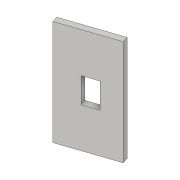
# Autodesk Inventor part: Lidar Sensor Case Piece 4
Saved by Autodesk Inventor 2018.3 (Build 223284000, 284)
## iProperties
Created: 2019-02-26
Part Number: Lidar Sensor Case Piece 4
Material: Generic
Document SubType Name: Modeling
Designer: aye06091
Mass: 4.13207 g
Surface Area: 33.6312 cm^2
Volume: 4.13207 cm^3
Density: 1 g/cm^3
Appearance: Default
Author: aye06091
Autodesk Inventor part; units mm, degrees
ref_plane "YZ Plane" through (0, 0, 0) normal (1, 0, 0) x (0, 1, 0)
ref_plane "XZ Plane" through (0, 0, 0) normal (0, 1, 0) x (-1, 0, 0)
ref_plane "XY Plane" through (0, 0, 0) normal (0, 0, 1) x (1, 0, 0)
sketch "Sketch1" plane through (0, 0, 0) normal (0, 1, 0) x (-1, 0, 0)
  line L0 (1.0684, 9.7831) -> (-25.4217, 0.8993)
  line L1 (-26.3747, 3.741) -> (0.1154, 12.6248)
  line L2 (1.0684, 9.7831) -> (0.1154, 12.6248)
  line L3 (-25.4217, 0.8993) -> (-26.3747, 3.741)
  point P0 (0, 0)
  point P1 (-9.2456, 5.0352)
  dimension "d0" = 27.94
  dimension "d5" = 2.9972
  constraints: 8 end point
  measures "d0" distance of L0.start L0.end
  measures "d5" distance between parallel lines of L1 L0
extrude "Extrusion1" add sketch "Sketch1" along normal blind 52.8066
sketch "Sketch2" plane through (-1.0684, 0, 9.7831) normal (-0.318, 0, -0.9481) x (-0.9481, 0, 0.318)
  line L0 (0, 0) -> (-27.94, 0) projected
  line L1 (-27.94, 52.8066) -> (0, 52.8066) projected
  line L2 (-18.7775, 20.0533) -> (-11.1575, 20.0533)
  line L3 (-11.1575, 20.0533) -> (-11.1575, 32.7533)
  line L4 (-11.1575, 32.7533) -> (-18.7775, 32.7533)
  line L5 (-18.7775, 32.7533) -> (-18.7775, 20.0533)
  line L6 (0, 0) -> (0, 52.8066) projected
  point P0 (-4.1236, 0)
  dimension "d9" = 12.7
  dimension "d10" = 7.62
  dimension "d13" = 20.0533
  dimension "d14" = 20.0533
  dimension "d18" = 18.7775
  constraints: 8 end point, 2 parallel, 1 horizontal, 1 perpendicular
  measures "d9" distance of L4.end L2.start
  measures "d10" distance of L3.end L4.end
  measures "d13" distance between parallel lines of L1 L4
  measures "d14" distance between parallel lines of L0 L2
  measures "d18" distance between parallel lines of L6 L5
extrude "Extrusion2" cut sketch "Sketch2" against normal blind 25.4
body "Solid1"
